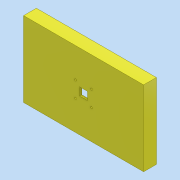
# Autodesk Inventor part: touchscreen_case
Saved by Autodesk Inventor 2022 (Build 260153000, 153)
## iProperties
Created: 2020-11-06
Part Number: touchscreen_case
Material: Generic
Document SubType Name: Modeling
Designer: nnico
Density: 1 g/cm^3
Appearance: Yellow
Author: nnico
Autodesk Inventor part; units mm, degrees
ref_plane "YZ Plane" through (0, 0, 0) normal (1, 0, 0) x (0, 1, 0)
ref_plane "XZ Plane" through (0, 0, 0) normal (0, 1, 0) x (-1, 0, 0)
ref_plane "XY Plane" through (0, 0, 0) normal (0, 0, 1) x (1, 0, 0)
sketch "Sketch1" plane through (0, 0, 0) normal (0, 1, 0) x (-1, 0, 0)
  line L0 (112.75, -70.75) -> (-112.75, -70.75)
  line L1 (-112.75, -70.75) -> (-112.75, 70.75)
  line L2 (-112.75, 70.75) -> (112.75, 70.75)
  line L3 (112.75, 70.75) -> (112.75, -70.75)
  line L4 (0, -70.75) -> (0, 70.75) construction
  line L5 (112.75, 0) -> (-112.75, 0) construction
  line L6 (112.75, -70.75) -> (102.75, -70.75)
  line L7 (102.75, -66.75) -> (102.75, -60.75)
  line L8 (102.75, -60.75) -> (108.75, -60.75)
  line L9 (112.75, -60.75) -> (112.75, -70.75)
  line L10 (112.75, 70.75) -> (102.75, 70.75)
  line L11 (102.75, 66.75) -> (102.75, 60.75)
  line L12 (102.75, 60.75) -> (108.75, 60.75)
  line L13 (112.75, 60.75) -> (112.75, 70.75)
  line L14 (-112.75, -70.75) -> (-102.75, -70.75)
  line L15 (-102.75, -66.75) -> (-102.75, -60.75)
  line L16 (-102.75, -60.75) -> (-108.75, -60.75)
  line L17 (-112.75, -60.75) -> (-112.75, -70.75)
  line L18 (-102.75, 60.75) -> (-108.75, 60.75)
  line L19 (-112.75, 60.75) -> (-112.75, 70.75)
  line L20 (-112.75, 70.75) -> (-102.75, 70.75)
  line L21 (-102.75, 66.75) -> (-102.75, 60.75)
  line L22 (102.75, -66.75) -> (-102.75, -66.75)
  line L23 (-108.75, -60.75) -> (-108.75, 60.75)
  line L24 (-102.75, 66.75) -> (102.75, 66.75)
  line L25 (108.75, 60.75) -> (108.75, -60.75)
  point P0 (0, 0)
  point P1 (0, 0)
  dimension "d0" = 225.5
  dimension "d1" = 141.5
  dimension "d2" = 10
  dimension "d3" = 10
  dimension "d5" = 4
  dimension "d6" = 4
  constraints: 52 end point, 9 symmetric about line, 6 parallel, 5 midpoint, 3 horizontal, 3 perpendicular, 1 coincident, 2 other
  measures "d0" distance of L0.start L0.end
  measures "d1" distance of L2.end L0.start
  measures "d2" distance of L7.end L9.start
  measures "d3" distance of L6.end L7.end
  measures "d5" distance between parallel lines of L25 L3
  measures "d6" distance between parallel lines of L0 L22
extrude "Extrusion1" add sketch "Sketch1" along normal blind 24
sketch "Sketch2" plane through (0, 24, 0) normal (0, 1, 0) x (1, 0, 0)
  line L0 (-108.75, 60.75) -> (-102.75, 60.75) construction
  line L1 (-102.75, 60.75) -> (-112.75, 60.75) construction
  line L2 (-112.75, 60.75) -> (-112.75, 70.75) construction
  line L3 (-112.75, 70.75) -> (-102.75, 70.75) construction
  line L4 (-102.75, 70.75) -> (-102.75, 60.75) construction
  line L5 (-112.75, 70.75) -> (-112.75, -70.75) construction
  line L6 (-112.75, 0) -> (112.75, 0) construction
  line L7 (112.75, 70.75) -> (112.75, -70.75) construction
  line L8 (-112.75, -70.75) -> (112.75, -70.75) construction
  line L9 (0, -70.75) -> (0, 70.75) construction
  line L10 (-112.75, 70.75) -> (112.75, 70.75) construction
  circle A0 centre (-107.75, 65.75) radius 2.75
  circle A1 centre (-107.75, -65.75) radius 2.75
  circle A2 centre (107.75, 65.75) radius 2.75
  circle A3 centre (107.75, -65.75) radius 2.75
  point P0 (0, 0)
  dimension "d9" = 5.5
  constraints: 12 end point, 4 centre point, 4 midpoint, 3 symmetric about line, 2 parallel, 1 horizontal, 1 perpendicular, 3 other
  measures "d9" diameter of A0
extrude "Extrusion2" cut sketch "Sketch2" against normal blind 7
sketch "Sketch4" plane through (0, 0, 0) normal (0, -1, 0) x (1, 0, 0)
  line L0 (-108.75, -60.75) -> (-108.75, 60.75) projected
  line L1 (-108.75, 60.75) -> (-102.75, 60.75) projected
  line L2 (-102.75, 60.75) -> (-102.75, 66.75) projected
  line L3 (-102.75, 66.75) -> (102.75, 66.75) projected
  line L4 (102.75, -66.75) -> (-102.75, -66.75) projected
  line L5 (-102.75, -66.75) -> (-102.75, -60.75) projected
  line L6 (-102.75, -60.75) -> (-108.75, -60.75) projected
  line L7 (102.75, -60.75) -> (102.75, -66.75) projected
  line L8 (108.75, -60.75) -> (102.75, -60.75) projected
  line L9 (108.75, 60.75) -> (108.75, -60.75) projected
  line L10 (102.75, 60.75) -> (108.75, 60.75) projected
  line L11 (102.75, 66.75) -> (102.75, 60.75) projected
  point P0 (0, 0)
extrude "Extrusion4" add sketch "Sketch4" against normal blind 4
sketch "Sketch5" plane through (0, 0, 0) normal (0, -1, 0) x (1, 0, 0)
  line L0 (112.75, -70.75) -> (-112.75, -70.75) construction
  line L1 (0, -70.75) -> (0, 70.75) construction
  line L2 (-112.75, 70.75) -> (112.75, 70.75) construction
  line L3 (112.75, 70.75) -> (112.75, -70.75) construction
  line L4 (112.75, 0) -> (-112.75, 0) construction
  line L5 (-112.75, -70.75) -> (-112.75, 70.75) construction
  line L6 (0, 0) -> (15, 0) construction
  line L7 (15, 0) -> (15, -15) construction
  line L8 (15, -15) -> (0, -15) construction
  line L9 (0, -15) -> (0, 0) construction
  circle A0 centre (15, -15) radius 1.75
  circle A1 centre (-15, -15) radius 1.75
  circle A2 centre (15, 15) radius 1.75
  circle A3 centre (-15, 15) radius 1.75
  line L10 (7.5, -7.5) -> (-7.5, -7.5)
  line L11 (-7.5, -7.5) -> (-7.5, 7.5)
  line L12 (-7.5, 7.5) -> (7.5, 7.5)
  line L13 (7.5, 7.5) -> (7.5, -7.5)
  dimension "d16" = 15
  dimension "d17" = 15
  dimension "d18" = 3.5
  dimension "d21" = 15
  dimension "d22" = 15
  dimension "d23" = 7.5
  dimension "d24" = 7.5
  constraints: 20 end point, 4 centre point, 4 midpoint, 4 parallel, 3 symmetric about line, 2 horizontal, 2 perpendicular, 1 coincident, 3 other
  measures "d16" distance of L7.end L8.end
  measures "d17" distance of L6.end L7.end
  measures "d18" diameter of A0
  measures "d21" distance of L11.end L12.end
  measures "d22" distance of L10.end L11.end
  measures "d23" distance from line of L10 L6.start
  measures "d24" distance from line of L6.start L13
extrude "Extrusion5" cut sketch "Sketch5" against normal up to next
body "Solid1"
